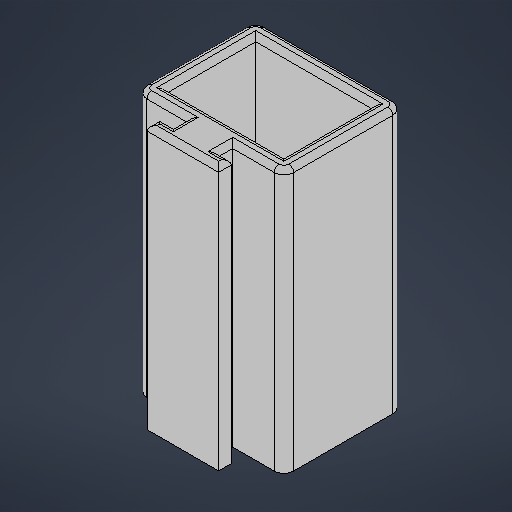
# Autodesk Inventor part: cajaBuck
Saved by Autodesk Inventor 2026.2 (Build 302298010, 298A)
## iProperties
Created: 2026-08-20
Part Number: cajaBuck
Material: Genérico
Document SubType Name: Modeling
Designer: samue
Density: 1 g/cm^3
Appearance: Valor por defecto
Author: samue
Autodesk Inventor part; units mm, degrees
ref_plane "YZ Plane" through (0, 0, 0) normal (1, 0, 0) x (0, 1, 0)
ref_plane "XZ Plane" through (0, 0, 0) normal (0, 1, 0) x (-1, 0, 0)
ref_plane "XY Plane" through (0, 0, 0) normal (0, 0, 1) x (1, 0, 0)
sketch "Boceto1" plane through (0, 0, 0) normal (0, 1, 0) x (-1, 0, 0)
  line L0 (0, 0) -> (0, -2.6)
  line L1 (0, -2.6) -> (-2.7, -2.6)
  line L2 (-2.7, -2.6) -> (-2.7, -5.7)
  line L3 (-2.7, -5.7) -> (-12, -5.7)
  line L4 (-12, -5.7) -> (-12, -2.6)
  line L5 (-12, -2.6) -> (-14.7, -2.6)
  line L6 (-14.7, -2.6) -> (-14.7, 0)
  line L7 (-14.7, 0) -> (0, 0)
  line L8 (-12, -5.7) -> (-11.9, -5.7)
  line L9 (-11.9, -5.7) -> (-11.9, -2.6)
  line L10 (-11.9, -2.6) -> (-12, -2.6)
  line L11 (-12, -2.6) -> (-12, -5.7)
  line L12 (-2.7, -5.7) -> (-2.8, -5.7)
  line L13 (-2.8, -5.7) -> (-2.8, -2.6)
  line L14 (-2.8, -2.6) -> (-2.7, -2.6)
  line L15 (-2.7, -2.6) -> (-2.7, -5.7)
  line L16 (-2.7, -5.7) -> (4.75, -5.7)
  line L17 (-2.7, -5.7) -> (4.75, -5.7) construction
  line L18 (-12, -5.7) -> (-19.45, -5.7)
  line L19 (-12, -5.7) -> (-4.55, -5.7) construction
  line L20 (4.75, -5.7) -> (5.75, -5.7)
  line L21 (7.75, -7.7) -> (7.75, -8.7)
  line L22 (7.75, -8.7) -> (4.75, -8.7)
  line L23 (4.75, -8.7) -> (4.75, -5.7)
  line L24 (-19.45, -5.7) -> (-20.45, -5.7)
  line L25 (-22.45, -7.7) -> (-22.45, -8.7)
  line L26 (-22.45, -8.7) -> (-19.45, -8.7)
  line L27 (-19.45, -8.7) -> (-19.45, -5.7)
  line L28 (4.75, -8.7) -> (-19.45, -8.7)
  line L29 (4.75, -8.7) -> (7.75, -8.7)
  line L30 (7.75, -8.7) -> (7.75, -27.1)
  line L31 (7.75, -27.1) -> (4.75, -27.1)
  line L32 (4.75, -27.1) -> (4.75, -8.7)
  line L33 (-22.45, -8.7) -> (-19.45, -8.7)
  line L34 (-19.45, -8.7) -> (-19.45, -27.1)
  line L35 (-19.45, -27.1) -> (-22.45, -27.1)
  line L36 (-22.45, -27.1) -> (-22.45, -8.7)
  line L37 (7.75, -27.1) -> (-22.45, -27.1)
  line L38 (-22.45, -27.1) -> (-22.45, -28.1)
  line L39 (-20.45, -30.1) -> (5.75, -30.1)
  line L40 (7.75, -28.1) -> (7.75, -27.1)
  arc A0 (7.75, -7.7) -> (5.75, -5.7) centre (5.75, -7.7) ccw
  arc A1 (5.75, -30.1) -> (7.75, -28.1) centre (5.75, -28.1) ccw
  arc A2 (-22.45, -28.1) -> (-20.45, -30.1) centre (-20.45, -28.1) ccw
  arc A3 (-20.45, -5.7) -> (-22.45, -7.7) centre (-20.45, -7.7) ccw
  point P0 (-7.35, -5.7)
  point P1 (7.75, -5.7)
  point P2 (-22.45, -5.7)
  point P3 (-22.45, -30.1)
  point P4 (7.75, -30.1)
  dimension "d0" = 2.6
  dimension "d1" = 2.7
  dimension "d2" = 3.1
  dimension "d3" = 2.7
  dimension "d4" = 9.3
  dimension "d5" = 0.1
  dimension "d6" = 0.1
  dimension "d7" = 0
  dimension "d8" = 12.1
  dimension "d9" = 180
  dimension "d10" = 12.1
  dimension "d11" = 3
  dimension "d12" = 3
  dimension "d13" = 3
  dimension "d14" = 3
  dimension "d15" = 18.4
  dimension "d16" = 3
  dimension "d17" = 3
  dimension "d18" = 3
  dimension "d19" = 30.2
  dimension "d20" = 2
  constraints: 82 end point, 14 parallel, 13 point on line, 12 perpendicular, 10 horizontal, 8 point on circle, 8 tangent, 4 centre point, 3 equal radius, 2 collinear, 1 midpoint, 1 vertical
  measures "d0" distance of L0.start L0.end
  measures "d1" distance of L0.end L1.end
  measures "d2" distance of L1.end L2.end
  measures "d3" distance of L4.end L5.end
  measures "d4" distance of L2.end L3.end
  measures "d5" distance of L10.end L9.end
  measures "d6" distance of L13.end L14.end
  measures "d7" distance between parallel lines of L16 L17
  measures "d8" distance of point (-7.35, -5.7) L16.end
  measures "d9" angle of L18 L19
  measures "d10" distance of point (-7.35, -5.7) L18.end
  measures "d11" distance of L21.end L22.end
  measures "d12" distance of point (7.75, -5.7) L21.end
  measures "d13" distance of L26.end L25.end
  measures "d14" distance of L25.end point (-22.45, -5.7)
  measures "d15" distance of L29.end L30.end
  measures "d16" distance of L30.end L31.end
  measures "d17" distance of L34.end L35.end
  measures "d18" distance of point (-22.45, -30.1) L37.end
  measures "d19" distance of point (-22.45, -30.1) point (7.75, -30.1)
  measures "d20" radius of A0
extrude "Extrusión1" add sketch "Boceto1" along normal blind 54.2 contours L0 L1 L14 L13 L3 L9 L10 L5 L6 L7 | L16 L23 L28 L27 L18 L3 | L20 A0 L21 L22 L23 | L22 L30 L31 L32 | L27 L26 L25 A3 L24 | L34 L35 L36 L26 | L31 L40 A1 L39 A2 L38 L35 L37
fillet "Empalme1" radius 1 20 edges at (-4.75, 54.2, -17.9) (-7.1642, 54.2, -29.5142) (-7.75, 54.2, -8.2) (-7.1642, 54.2, -6.2858) (2.75, 54.2, -5.7) (21.8642, 54.2, -29.5142) (22.45, 54.2, -8.2) (21.8642, 54.2, -6.2858) (11.95, 54.2, -5.7) (7.35, 54.2, -30.1) (7.35, 54.2, -27.1) (19.45, 54.2, -17.9) (7.35, 54.2, -8.7) (11.9, 54.2, -4.15) (2.8, 54.2, -4.15) (1.35, 54.2, -2.6) (0, 54.2, -1.3) (7.35, 54.2, 0) (14.7, 54.2, -1.3) (13.35, 54.2, -2.6)
